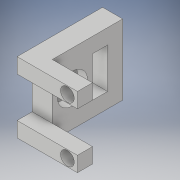
# Autodesk Inventor part: TensionerPlate
Saved by Autodesk Inventor 2017 (Build 210142000, 142)
## iProperties
Created: 2017-07-29
Part Number: TensionerPlate
Material: Generic
Document SubType Name: Modeling
Designer: User
Density: 1 g/cm^3
Appearance: Default
Author: User
Autodesk Inventor part; units mm, degrees
ref_plane "YZ Plane" through (0, 0, 0) normal (1, 0, 0) x (0, 1, 0)
ref_plane "XZ Plane" through (0, 0, 0) normal (0, 1, 0) x (-1, 0, 0)
ref_plane "XY Plane" through (0, 0, 0) normal (0, 0, 1) x (1, 0, 0)
sketch "Sketch1" plane through (0, 0, 0) normal (1, 0, 0) x (0, 1, 0)
  line L0 (22.225, 0) -> (22.225, -26.9875)
  line L1 (22.225, -26.9875) -> (0, -26.9875)
  line L2 (0, -26.9875) -> (0, 0)
  line L3 (17.4625, 0) -> (17.4625, -4.7625)
  line L4 (17.4625, -4.7625) -> (4.7625, -4.7625)
  line L5 (4.7625, -4.7625) -> (4.7625, 0)
  line L6 (6.35, -26.9875) -> (25.4, -26.9875)
  line L7 (0, 0) -> (4.7625, 0)
  line L8 (17.4625, 0) -> (22.225, 0)
  line L9 (4.7625, -17.4625) -> (17.4625, -17.4625)
  line L10 (17.4625, -17.4625) -> (17.4625, -22.225)
  line L11 (17.4625, -22.225) -> (4.7625, -22.225)
  line L12 (4.7625, -22.225) -> (4.7625, -17.4625)
  dimension "d6" = 4.7625
  dimension "d8" = 12.7
  dimension "d9" = 4.7625
  dimension "d10" = 4.7625
  dimension "d11" = 4.7625
  dimension "d27" = 4.7625
  dimension "d28" = 4.7625
  dimension "d29" = 4.7625
  dimension "d37" = 26.9875
  dimension "d38" = 26.9875
  constraints: 26 end point, 6 parallel, 4 horizontal, 3 perpendicular, 1 point on line
  measures "d6" distance between parallel lines of L2 L5
  measures "d8" distance of L10.end L11.end
  measures "d9" distance of L9.end L10.end
  measures "d10" distance between parallel lines of L1 L11
  measures "d11" distance between parallel lines of L2 L12
  measures "d27" distance between parallel lines of L3 L0
  measures "d28" distance between parallel lines of L10 L0
  measures "d29" distance of L3.start L3.end
  measures "d37" distance of L0.start L0.end
  measures "d38" distance of L1.end L2.end
extrude "Extrusion1" add sketch "Sketch1" along normal blind 6.35
sketch "Sketch2" plane through (6.35, 0, 0) normal (1, 0, 0) x (0, 0, -1)
  line L0 (17.4625, 17.4625) -> (22.225, 17.4625) projected
  line L1 (22.225, 17.4625) -> (22.225, 4.7625) projected
  line L2 (22.225, 4.7625) -> (17.4625, 4.7625) projected
  line L3 (17.4625, 4.7625) -> (17.4625, 17.4625) projected
  line L4 (0, 0) -> (26.9875, 0) projected
  line L5 (26.9875, 0) -> (26.9875, 22.225) projected
  line L6 (26.9875, 22.225) -> (0, 22.225) projected
  line L7 (0, 22.225) -> (0, 17.4625) projected
  line L8 (0, 17.4625) -> (4.7625, 17.4625) projected
  line L9 (4.7625, 17.4625) -> (4.7625, 4.7625) projected
  line L10 (4.7625, 4.7625) -> (0, 4.7625) projected
  line L11 (0, 4.7625) -> (0, 0) projected
  circle A0 centre (11.1125, 11.1125) radius 4.7625
  dimension "d14" = 9.525
  dimension "d15" = 11.1125
  dimension "d16" = 6.35
  dimension "d39" = 22.225
  constraints: 1 centre point
  measures "d14" diameter of A0
  measures "d15" distance from line of L6 A0.centre
  measures "d16" distance from line of L9 A0.centre
  measures "d39" distance of L4.end L5.end
extrude "Extrusion2" cut sketch "Sketch2" against normal blind 3.175 contours A0
sketch "Sketch3" plane through (0, 17.4625, 0) normal (0, 0, 1) x (1, 0, 0)
  line L0 (0, 4.7625) -> (0, 0) projected
  line L1 (0, 0) -> (6.35, 0) projected
  line L2 (6.35, 4.7625) -> (6.35, 0) projected
  line L3 (0, 4.7625) -> (6.35, 4.7625) projected
  line L4 (0, -12.7) -> (0, -17.4625) projected
  line L5 (0, -17.4625) -> (6.35, -17.4625) projected
  line L6 (6.35, -12.7) -> (6.35, -17.4625) projected
  line L7 (0, -12.7) -> (6.35, -12.7) projected
  line L8 (0, 4.7625) -> (19.05, 4.7625)
  line L9 (19.05, 4.7625) -> (19.05, 0)
  line L10 (19.05, 0) -> (0, 0)
  line L11 (0, 0) -> (0, 4.7625)
  circle A0 centre (15.875, 2.3812) radius 2.159
  circle A1 centre (15.875, -15.0812) radius 2.159
  line L12 (0, -17.4625) -> (19.05, -17.4625)
  line L13 (19.05, -17.4625) -> (19.05, -12.7)
  line L14 (19.05, -12.7) -> (0, -12.7)
  line L15 (0, -12.7) -> (0, -17.4625)
  dimension "d21" = 19.05
  dimension "d22" = 4.318
  dimension "d23" = 3.175
  dimension "d24" = 4.318
  dimension "d30" = 0
  dimension "d31" = 4.7625
  dimension "d32" = 2.3813
  dimension "d33" = 19.05
  dimension "d34" = 2.3813
  dimension "d35" = 3.175
  constraints: 16 end point, 4 parallel, 2 centre point, 2 horizontal, 2 perpendicular
  measures "d21" distance of L9.end L10.end
  measures "d22" diameter of A0
  measures "d23" distance from line of L9 A0.centre
  measures "d24" diameter of A1
  measures "d30" distance between parallel lines of L1 L10
  measures "d31" distance of L8.end L9.end
  measures "d32" distance from line of L10 A0.centre
  measures "d33" distance of L14.end L13.end
  measures "d34" distance from line of L14 A1.centre
  measures "d35" distance from line of L13 A1.centre
extrude "Extrusion3" add sketch "Sketch3" against normal blind 4.7625 contours L8 L9 L10 L2 | L14 L13 L12 L6
sketch "Sketch4" plane through (6.35, 0, 0) normal (1, 0, 0) x (0, 0, -1)
  line L0 (4.7625, 22.225) -> (4.7625, 17.4625) projected
  line L1 (4.7625, 17.4625) -> (4.7625, 4.7625) projected
  line L2 (4.7625, 4.7625) -> (4.7625, 0) projected
  line L3 (4.7625, 0) -> (26.9875, 0) projected
  line L4 (26.9875, 0) -> (26.9875, 22.225) projected
  line L5 (26.9875, 22.225) -> (4.7625, 22.225) projected
  line L6 (17.4625, 17.4625) -> (22.225, 17.4625) projected
  line L7 (22.225, 17.4625) -> (22.225, 4.7625) projected
  line L8 (22.225, 4.7625) -> (17.4625, 4.7625) projected
  line L9 (17.4625, 4.7625) -> (17.4625, 17.4625) projected
  circle A0 centre (11.1125, 11.1125) radius 4.7625 projected
  circle A1 centre (11.1125, 11.1125) radius 1.5875
  point P0 (0, 0)
  dimension "d40" = 3.175
  constraints: 1 centre point, 1 coincident
  measures "d40" diameter of A1
extrude "Extrusion4" cut sketch "Sketch4" against normal blind 25.4 contours A1
equation "\"d38\" = d37"
equation "\"d15\" = 0.5 * d39"
equation "\"d32\" = 0.5 * d31"
equation "\"d34\" = d32"
equation "\"d35\" = d23"
body "Solid1"
